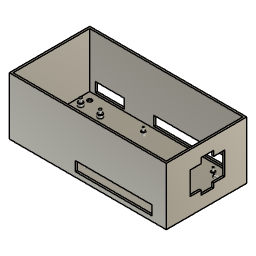
Gehäuse Filamentschrank (Autodesk Fusion 360 design; units mm, degrees)
Autodesk Fusion 360 part; units mm, degrees
sketch "Skizze1" plane through (0, 0, 0) normal (0, 0, 1) x (1, 0, 0)
  line L0 (0, 0) -> (160, 0)
  line L1 (160, 0) -> (160, 80)
  line L2 (160, 80) -> (0, 80)
  line L3 (0, 80) -> (0, 0)
  circle A0 centre (140, 10) radius 0.9
  line L4 (140, 10) -> (140, 69)
  circle A1 centre (140, 69) radius 0.9
  line L5 (140, 69) -> (67, 69)
  circle A2 centre (67, 69) radius 0.9
  circle A3 centre (67, 10) radius 0.9
  line L6 (140, 10) -> (67, 10)
  circle A4 centre (67, 69) radius 2
  circle A5 centre (67, 10) radius 2
  circle A6 centre (140, 10) radius 2
  circle A7 centre (140, 69) radius 2
  line L7 (-2, -2) -> (162, -2)
  line L8 (162, -2) -> (162, 82)
  line L9 (162, 82) -> (-2, 82)
  line L10 (-2, 82) -> (-2, -2)
  line L11 (8, 18) -> (8, 62.5)
  line L12 (28.5, 18) -> (28.5, 62.5)
  line L13 (28.5, 18) -> (8, 18)
  circle A8 centre (28.5, 18) radius 2.5
  circle A9 centre (28.5, 18) radius 1.375
  circle A10 centre (8, 18) radius 2.5
  circle A11 centre (8, 18) radius 1.375
  circle A12 centre (8, 62.5) radius 1.375
  circle A13 centre (8, 62.5) radius 2.5
  circle A14 centre (28.5, 62.5) radius 2.5
  circle A15 centre (28.5, 62.5) radius 1.375
  dimension "d1" = 160
  dimension "d2" = 80
  dimension "d5" = 1.8
  dimension "d6" = 59
  dimension "d7" = 1.8
  dimension "d8" = 73
  dimension "d9" = 1.8
  dimension "d10" = 1.8
  dimension "d11" = 20
  dimension "d12" = 73
  dimension "d34" = 4
  dimension "d37" = 4
  dimension "d38" = 4
  dimension "d39" = 4
  dimension "d58" = 2
  dimension "d96" = 2.75
  dimension "d97" = 44.5
  dimension "d98" = 20.5
  dimension "d99" = 2.75
  dimension "d100" = 2.75
  dimension "d101" = 2.75
  dimension "d102" = 44.5
  dimension "d103" = 5
  dimension "d104" = 5
  dimension "d105" = 5
  dimension "d106" = 5
  dimension "d107" = 8
  dimension "d108" = 18
  constraint horizontal L0
  constraint vertical L1
  constraint horizontal L2
  constraint vertical L3
  constraint coincident L0.start L3.end
  constraint coincident A0.centre L4.start
  constraint vertical L4
  constraint coincident L4.end A1.centre
  constraint perpendicular L4 L5
  constraint coincident L5.end A2.centre
  constraint coincident A3.centre L6.end
  constraint perpendicular L4 L6
  constraint concentric A2 A4
  constraint concentric A0 A6
  constraint coincident L12.start L13.start
  constraint perpendicular L12 L13
  constraint coincident L12.end A14.centre
  constraint coincident L11.start L13.end
  constraint perpendicular L11 L13
  constraint coincident L11.end A12.centre
  constraint concentric A12 A13
  constraint concentric A8 A9
  measures "d1" distance of L0.start L0.end
  measures "d2" distance of L0.start L2.end
  measures "d5" diameter of A0
  measures "d6" distance of A0.centre L4.end
  measures "d7" diameter of A1
  measures "d8" distance of L4.end L5.end
  measures "d9" diameter of A2
  measures "d10" diameter of A3
  measures "d11" distance of L1 L4.end
  measures "d12" distance of A0.centre A3.centre
  measures "d34" diameter of A4
  measures "d37" diameter of A5
  measures "d38" diameter of A6
  measures "d39" diameter of A7
  measures "d96" diameter of A9
  measures "d97" distance of L12.start L12.end
  measures "d98" distance of L11.start L12.start
  measures "d99" diameter of A15
  measures "d100" diameter of A11
  measures "d101" diameter of A12
  measures "d102" distance of L11.start L11.end
  measures "d103" diameter of A13
  measures "d104" diameter of A14
  measures "d105" diameter of A10
  measures "d106" diameter of A8
  measures "d107" distance of L3 L11
  measures "d108" distance of L0 L13
extrude "Extrusion1" add sketch "Skizze1" along normal blind 3 contours L0 L1 L2 L3 | A0 L4 L6 A6 | A0 L4 L6 A6 | L4 A1 L5 A7 | L4 A1 L5 A7 | A4 | A5 | L11 L13 A11 | L11 L13 A11 | L11 L13 A10 A11 | L11 L13 A10 A11 | L12 L13 A9 | L12 L13 A9 | L12 L13 A8 A9 | L12 L13 A8 A9 | A12 | A13 | A14 | A15 makes body 1
extrude "Extrusion2" add sketch "Skizze1" along normal blind 6 separate body contours A0 L4 L6 | A0 L4 L6 A6 | A0 L4 L6 | A0 L4 L6 A6 | L4 A1 L5 A7 | L4 A1 L5 A7 | L4 A1 L5 | L4 A1 L5 | A2 | A3 | A4 | A5 makes body 2 at (65.0618, 68.5065, 4) makes body 3 at (141.3234, 67.5004, 2) makes body 4 at (68.3234, 11.4996, 4) makes body 5 at (138.6035, 8.5683, 2)
extrude "Extrusion3" add sketch "Skizze1" along normal blind 4 from surface at 6 contours A0 L4 L6 | A0 L4 L6 | L4 A1 L5 | L4 A1 L5 | A2 | A3 bodies 2 3 4 5
sketch "Skizze2" plane through (0, 0, 3) normal (0, 0, 1) x (-1, 0, 0)
  circle A0 centre (-140, -10) radius 0.9
  circle A1 centre (-140, -69) radius 0.9
  circle A2 centre (-67, -69) radius 0.9
  circle A3 centre (-67, -10) radius 0.9
  line L0 (0, -80) -> (0, 0)
  line L1 (0, 0) -> (-160, 0)
  line L2 (-160, 0) -> (-160, -80)
  line L3 (-160, -80) -> (0, -80)
  line L4 (0, -80) -> (-8, -80)
  line L5 (-8, -80) -> (-8, -72)
  line L6 (-8, -72) -> (0, -72)
  line L7 (0, -72) -> (0, -80)
  line L8 (0, 0) -> (-8, 0)
  line L9 (-8, 0) -> (-8, -8)
  line L10 (-8, -8) -> (0, -8)
  line L11 (0, -8) -> (0, 0)
  line L12 (-160, 0) -> (-152, 0)
  line L13 (-152, 0) -> (-152, -8)
  line L14 (-152, -8) -> (-160, -8)
  line L15 (-160, -8) -> (-160, 0)
  line L16 (-160, -80) -> (-152, -80)
  line L17 (-152, -80) -> (-152, -72)
  line L18 (-152, -72) -> (-160, -72)
  line L19 (-160, -72) -> (-160, -80)
  dimension "d45" = 8
  dimension "d46" = 8
  dimension "d47" = 8
  dimension "d48" = 8
  dimension "d49" = 8
  dimension "d50" = 8
  dimension "d51" = 8
  dimension "d52" = 8
  constraint horizontal L4
  constraint vertical L5
  constraint horizontal L6
  constraint vertical L7
  constraint coincident L0.start L3.end
  constraint horizontal L8
  constraint vertical L9
  constraint horizontal L10
  constraint vertical L11
  constraint coincident L0.end L1.start
  constraint horizontal L12
  constraint vertical L13
  constraint horizontal L14
  constraint vertical L15
  constraint coincident L1.end L2.start
  constraint horizontal L16
  constraint vertical L17
  constraint horizontal L18
  constraint vertical L19
  constraint coincident L2.end L3.start
  measures "d45" distance of L0.start L4.end
  measures "d46" distance of L0.start L6.end
  measures "d47" distance of L0.end L8.end
  measures "d48" distance of L0.end L10.end
  measures "d49" distance of L1.end L12.end
  measures "d50" distance of L1.end L14.end
  measures "d51" distance of L2.end L16.end
  measures "d52" distance of L2.end L18.end
hole "Bohrung1" at (8, 72, 3) at (8, 8, 3) at (152, 8, 3) at (152, 72, 3) direction (0, 0, -1) diameter 3 depth 3 tip angle 180 countersink diameter 4.5 countersink angle 90 bodies 1
extrude "Extrusion4" add sketch "Skizze1" along normal blind 60 contours L7 L8 L9 L10 bodies 1
sketch "Skizze3" plane through (162, 0, 0) normal (1, 0, 0) x (0, 1, 0)
  line L0 (-2, 0) -> (82, 0)
  line L1 (82, 0) -> (82, 60)
  line L2 (82, 60) -> (-2, 60)
  line L3 (-2, 60) -> (-2, 0)
  line L4 (23, 47) -> (23, 13)
  line L5 (23, 13) -> (59, 13)
  line L6 (59, 13) -> (59, 47)
  line L7 (59, 47) -> (23, 47)
  line L8 (-2, 0) -> (82, 0)
  line L9 (0, 3) -> (0, 60)
  circle A0 centre (25.5, 44.35) radius 1.45
  circle A1 centre (25.5, 15.65) radius 1.45
  circle A2 centre (56, 44.35) radius 1.45
  circle A3 centre (56, 15.65) radius 1.45
  line L10 (23, 17.5) -> (23, 40.5)
  line L11 (23, 40.5) -> (59, 40.5)
  line L12 (59, 40.5) -> (59, 17.5)
  line L13 (59, 17.5) -> (23, 17.5)
  line L14 (47.5, 17.5) -> (47.5, 13)
  line L15 (47.5, 13) -> (34.5, 13)
  line L16 (34.5, 13) -> (34.5, 17.5)
  line L17 (34.5, 17.5) -> (47.5, 17.5)
  line L18 (47.5, 47) -> (47.5, 44)
  line L19 (47.5, 44) -> (34.5, 44)
  line L20 (34.5, 44) -> (34.5, 47)
  line L21 (34.5, 47) -> (47.5, 47)
  line L22 (34.5, 44) -> (47.5, 44)
  line L23 (47.5, 44) -> (47.5, 40.5)
  line L24 (47.5, 40.5) -> (34.5, 40.5)
  line L25 (34.5, 40.5) -> (34.5, 44)
  line L26 (23, 40.5) -> (59, 40.5)
  line L27 (59, 40.5) -> (59, 41.5)
  line L28 (59, 41.5) -> (23, 41.5)
  line L29 (23, 41.5) -> (23, 40.5)
  dimension "d62" = 34
  dimension "d63" = 36
  dimension "d69" = 2.9
  dimension "d70" = 2.5
  dimension "d71" = 2.65
  dimension "d72" = 2.9
  dimension "d73" = 2.9
  dimension "d74" = 2.9
  dimension "d75" = 3
  dimension "d76" = 3
  dimension "d77" = 2.5
  dimension "d78" = 2.65
  dimension "d79" = 2.65
  dimension "d80" = 2.65
  dimension "d81" = 4.5
  dimension "d82" = 23
  dimension "d87" = 13
  dimension "d88" = 11.5
  dimension "d91" = 3
  dimension "d92" = 13
  dimension "d93" = 11.5
  dimension "d117" = 13
  dimension "d118" = 23
  dimension "d119" = 1
  constraint coincident L13 L14.start
  constraint coincident L7 L18.start
  constraint horizontal L22
  constraint vertical L23
  constraint horizontal L24
  constraint vertical L25
  constraint coincident L11 L23.end
  constraint horizontal L26
  constraint vertical L27
  constraint horizontal L28
  constraint vertical L29
  measures "d62" distance of L4.start L4.end
  measures "d63" distance of L4.start L6.end
  measures "d69" diameter of A0
  measures "d70" distance of L4 A0.centre
  measures "d71" distance of L7 A0.centre
  measures "d72" diameter of A1
  measures "d73" diameter of A2
  measures "d74" diameter of A3
  measures "d75" distance of L6 A2.centre
  measures "d76" distance of L6 A3.centre
  measures "d77" distance of L4 A1.centre
  measures "d78" distance of L5 A1.centre
  measures "d79" distance of L5 A3.centre
  measures "d80" distance of L7 A2.centre
  measures "d81" distance of L4.end L10.start
  measures "d82" distance of L10.start L10.end
  measures "d87" distance of L14.start L16.end
  measures "d88" distance of L6 L14
  measures "d91" distance of L18.start L18.end
  measures "d92" distance of L18.start L20.end
  measures "d93" distance of L6 L18
  measures "d117" distance of L5 L8
  measures "d118" distance of L1 L6
  measures "d119" distance of L10.end L28.end
extrude "Extrusion5" add sketch "Skizze3" against normal blind 8 contours A0 | A1 | A2 | A3 bodies 1
extrude "Extrusion6" cut sketch "Skizze3" against normal blind 3 contours L4 L6 L10 L11 L12 L13 L17 L24 L26 bodies 1
extrude "Extrusion7" cut sketch "Skizze3" against normal blind 2 contours L5 L13 L14 L15 L16 L17 bodies 1
extrude "Extrusion8" cut sketch "Skizze3" against normal blind 2 contours L7 L18 L19 L20 L21 L22 bodies 1
extrude "Extrusion9" add sketch "Skizze1" along normal blind 6 contours L11 L13 A10 A11 | L11 L13 A10 A11 | L12 L13 A8 A9 | L12 L13 A8 A9 | A13 | A14 bodies 1
extrude "Extrusion10" add sketch "Skizze1" along normal blind 10 contours L11 L13 A11 | L11 L13 A11 | L12 L13 A9 | L12 L13 A9 | A12 | A15 bodies 1
extrude "Extrusion11" cut sketch "Skizze3" against normal blind 2 contours L4 L11 L25 L26 L28 L29 | L11 L23 L24 L25 L26 L28 | L19 L22 L23 L25 L28 | L6 L11 L23 L26 L27 L28 bodies 1
sketch "Skizze4" plane through (0, 82, 0) normal (0, 1, 0) x (-1, 0, 0)
  line L0 (-162, 0) -> (2, 0)
  line L1 (2, 0) -> (2, 60)
  line L2 (2, 60) -> (-162, 60)
  line L3 (-162, 60) -> (-162, 0)
  line L4 (-162, 0) -> (2, 0)
  line L5 (2, 0) -> (2, 5)
  line L6 (2, 5) -> (-162, 5)
  line L7 (-162, 5) -> (-162, 0)
  line L8 (-147, 5) -> (-67, 5)
  line L9 (-67, 5) -> (-67, 15)
  line L10 (-67, 15) -> (-147, 15)
  line L11 (-147, 15) -> (-147, 5)
  line L12 (-35.9542, 10) -> (-5.9542, 10)
  line L13 (-5.9542, 10) -> (-5.9542, 5)
  line L14 (-5.9542, 5) -> (-35.9542, 5)
  line L15 (-35.9542, 5) -> (-35.9542, 10)
  line L16 (-35.9542, 10) -> (-5.9542, 10)
  line L17 (-5.9542, 10) -> (-5.9542, 15)
  line L18 (-5.9542, 15) -> (-35.9542, 15)
  line L19 (-35.9542, 15) -> (-35.9542, 10)
  dimension "d122" = 5
  dimension "d123" = 80
  dimension "d124" = 10
  dimension "d125" = 30
  dimension "d128" = 5
  dimension "d129" = 5
  dimension "d138" = 15
  constraint horizontal L4
  constraint vertical L5
  constraint horizontal L6
  constraint vertical L7
  constraint coincident L0.start L3.end
  constraint horizontal L8
  constraint vertical L9
  constraint horizontal L10
  constraint vertical L11
  constraint coincident L6 L8.start
  constraint horizontal L12
  constraint vertical L13
  constraint horizontal L14
  constraint vertical L15
  constraint horizontal L16
  constraint vertical L17
  constraint horizontal L18
  constraint vertical L19
  measures "d122" distance of L0.start L6.end
  measures "d123" distance of L8.start L8.end
  measures "d124" distance of L8.start L10.end
  measures "d125" distance of L12.start L12.end
  measures "d128" distance of L12.start L14.end
  measures "d129" distance of L12.start L18.end
  measures "d138" distance of L3 L11
extrude "Extrusion12" cut sketch "Skizze4" against normal blind 2 contours L6 L8 L9 L10 L11 | L6 L12 L13 L14 L15 L16 bodies 1
extrude "Extrusion13" cut sketch "Skizze4" against normal blind 2 contours L12 L16 L17 L18 L19 bodies 1
sketch "Skizze5" plane through (0, -2, 0) normal (0, -1, 0) x (1, 0, 0)
  line L0 (-2, 0) -> (162, 0)
  line L1 (162, 0) -> (162, 60)
  line L2 (162, 60) -> (-2, 60)
  line L3 (-2, 60) -> (-2, 0)
  line L4 (-2, 0) -> (162, 0)
  line L5 (162, 0) -> (162, 5)
  line L6 (162, 5) -> (-2, 5)
  line L7 (-2, 5) -> (-2, 0)
  line L8 (147, 5) -> (67, 5)
  line L9 (67, 5) -> (67, 15)
  line L10 (67, 15) -> (147, 15)
  line L11 (147, 15) -> (147, 5)
  dimension "d132" = 5
  dimension "d133" = 80
  dimension "d134" = 10
  dimension "d137" = 15
  constraint horizontal L4
  constraint vertical L5
  constraint horizontal L6
  constraint vertical L7
  constraint coincident L0.start L3.end
  constraint horizontal L8
  constraint vertical L9
  constraint horizontal L10
  constraint vertical L11
  constraint coincident L6 L8.start
  measures "d132" distance of L0.start L6.end
  measures "d133" distance of L8.start L8.end
  measures "d134" distance of L8.start L10.end
  measures "d137" distance of L1 L11
extrude "Extrusion14" cut sketch "Skizze5" against normal blind 2 contours L6 L8 L9 L10 L11 bodies 1
equation "d71 = 1.45 mm + 1.2 mm"
